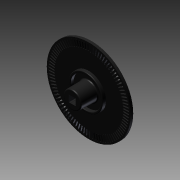
# Autodesk Inventor part: 276-2156
Saved by Autodesk Inventor 2013 (Build 170138000, 138)
## iProperties
Category: Sensors
Company: Autodesk Inc.
Created: 2012-04-06
Part Number: 276-2156
Document SubType Name: Modeling
Designer: Autodesk Inc.
Density: 1 g/cm^3
Catalog Web Link: http://www.vexrobotics.com/276-2156.html
Vendor: VEX
Material: Generic
Author: Autodesk Inc.
Autodesk Inventor part; units mm, degrees
ref_plane "YZ Plane" through (0, 0, 0) normal (1, 0, 0) x (0, 1, 0)
ref_plane "XZ Plane" through (0, 0, 0) normal (0, 1, 0) x (-1, 0, 0)
ref_plane "XY Plane" through (0, 0, 0) normal (0, 0, 1) x (1, 0, 0)
sketch "Sketch1" plane through (0, 0, 0) normal (0, 0, 1) x (1, 0, 0)
  circle A0 centre (0, 0) radius 20.0025
  dimension "d0" = 40.005
  constraints: 1 centre point, 1 coincident
  measures "d0" diameter of A0
extrude "Extrusion1" add sketch "Sketch1" along normal mid plane 1.2446
sketch "Sketch2" plane through (0, 0, 0.6223) normal (0, 0, 1) x (1, 0, 0)
  circle A0 centre (0, 0) radius 20.0025 projected
  circle A1 centre (0, 0) radius 4.3187
  dimension "d3" = 8.6374
  constraints: 1 centre point, 1 coincident
  measures "d3" diameter of A1
extrude "Extrusion2" add sketch "Sketch2" along normal blind 7.874 draft -0.5 contours A1
fillet "Fillet1" radius 0.508 2 edges at (-4.3187, 0, 0.6223) (-4.25, 0, 8.4963)
sketch "Sketch3" plane through (0, 0, 0.6223) normal (0, 0, 1) x (1, 0, 0)
  circle A0 centre (0, 0) radius 4.8223 projected
  circle A1 centre (0, 0) radius 7.2238
  circle A2 centre (0, 0) radius 8.2652
  dimension "d7" = 14.4476
  dimension "d8" = 1.0414
  constraints: 2 centre point, 2 coincident
  measures "d7" diameter of A1
  measures "d8" radial gap between concentric circles of A2 A1
extrude "Extrusion3" add sketch "Sketch3" along normal blind 1.4986 draft -1 contours A2
fillet "Fillet2" radius 0.3048 2 edges at (-8.2391, 0, 2.1209) (-7.25, 0, 2.1209)
mirror "Mirror1" about plane through (0, 0, 0) normal (0, 0, 1) of "Extrusion1", "Extrusion2", "Fillet1"
sketch "Sketch4" plane through (0, 0, 8.4963) normal (0, 0, 1) x (1, 0, 0)
  ellipse E0 centre (0.0646, -0.7293) end of major axis (-2.4878, -3.9719) minor radius 3.3908 (3.7543, 0.0005) -> (3.7536, 0.0771) ccw
  spline S0 degree 3 poles (3.7536, 0.0771) (3.7488, 0.3133) (3.7224, 0.5454) (3.6744, 0.7733) (3.6504, 0.8873) (3.6209, 1.0002) (3.5861, 1.1121) (3.5512, 1.224) (3.5122, 1.3325) (3.4637, 1.4484) (3.3668, 1.6803) (3.2489, 1.8987) (3.1046, 2.111) (2.9603, 2.3234) (2.7944, 2.5203) (2.6099, 2.6988) (2.5176, 2.7881) (2.4212, 2.8723) (2.3205, 2.9514) (2.2198, 3.0306) (2.1131, 3.1057) (2.0069, 3.1729) (1.9007, 3.2401) (1.7915, 3.3018) (1.6793, 3.3579) (1.6232, 3.3859) (1.5664, 3.4126) (1.5088, 3.4378) (1.4512, 3.4631) (1.3921, 3.4872) (1.3369, 3.5083) (1.116, 3.5926) (0.8909, 3.6552) (0.6616, 3.6962) (0.4323, 3.7372) (0.1977, 3.7565) (-0.0388, 3.7542) (-0.2753, 3.7518) (-0.5078, 3.7278) (-0.7362, 3.6821) (-0.8504, 3.6592) (-0.9635, 3.6309) (-1.0757, 3.5972) (-1.1318, 3.5804) (-1.1876, 3.5622) (-1.2432, 3.5426) (-1.2988, 3.523) (-1.3525, 3.5028) (-1.4108, 3.4792) (-1.5273, 3.432) (-1.6411, 3.3791) (-1.752, 3.3206) (-1.8629, 3.262) (-1.9695, 3.1988) (-2.0766, 3.1278) (-2.2906, 2.9857) (-2.4891, 2.8223) (-2.6698, 2.6396) (-2.7601, 2.5483) (-2.8454, 2.4527) (-2.9256, 2.3529) (-2.9658, 2.303) (-3.0046, 2.252) (-3.0422, 2.2) (-3.0798, 2.148) (-3.1168, 2.094) (-3.151, 2.0412) (-3.2194, 1.9356) (-3.2823, 1.827) (-3.3395, 1.7155) (-3.3682, 1.6597) (-3.3954, 1.6032) (-3.4213, 1.546) (-3.4342, 1.5173) (-3.4468, 1.4885) (-3.459, 1.4595) (-3.4713, 1.4305) (-3.4836, 1.4001) (-3.4945, 1.3725) (-3.6677, 0.9317) (-3.7543, 0.474) (-3.7543, -0.0005) knots 0.006695 0.006695 0.006695 0.006695 0.068777 0.068777 0.068777 0.099817 0.099817 0.099817 0.130858 0.130858 0.130858 0.19294 0.19294 0.19294 0.255021 0.255021 0.255021 0.286062 0.286062 0.286062 0.317103 0.317103 0.317103 0.348144 0.348144 0.348144 0.363664 0.363664 0.363664 0.379184 0.379184 0.379184 0.441266 0.441266 0.441266 0.503348 0.503348 0.503348 0.565429 0.565429 0.565429 0.59647 0.59647 0.59647 0.61199 0.61199 0.61199 0.627511 0.627511 0.627511 0.658551 0.658551 0.658551 0.689592 0.689592 0.689592 0.751674 0.751674 0.751674 0.782715 0.782715 0.782715 0.798235 0.798235 0.798235 0.813755 0.813755 0.813755 0.844796 0.844796 0.844796 0.860316 0.860316 0.860316 0.868077 0.868077 0.868077 0.875837 0.875837 0.875837 1 1 1 1
  arc A0 (-3.7543, -0.0005) -> (-3.7536, -0.0771) centre (0, 0) ccw
  spline S1 degree 3 poles (-3.7536, -0.0771) (-3.7488, -0.3133) (-3.7224, -0.5454) (-3.6744, -0.7733) (-3.6504, -0.8873) (-3.6209, -1.0002) (-3.5861, -1.1121) (-3.5512, -1.224) (-3.5122, -1.3324) (-3.4637, -1.4484) (-3.3668, -1.6803) (-3.2489, -1.8987) (-3.1046, -2.111) (-2.9603, -2.3234) (-2.7944, -2.5203) (-2.6099, -2.6988) (-2.5176, -2.7881) (-2.4212, -2.8723) (-2.3205, -2.9514) (-2.2198, -3.0306) (-2.1131, -3.1057) (-2.0069, -3.1729) (-1.9007, -3.2401) (-1.7915, -3.3018) (-1.6793, -3.3579) (-1.6232, -3.3859) (-1.5664, -3.4126) (-1.5088, -3.4378) (-1.4512, -3.4631) (-1.3921, -3.4872) (-1.3369, -3.5083) (-1.116, -3.5926) (-0.8909, -3.6552) (-0.6616, -3.6962) (-0.4323, -3.7372) (-0.1977, -3.7565) (0.0388, -3.7541) (0.2753, -3.7518) (0.5078, -3.7278) (0.7362, -3.6821) (0.8504, -3.6592) (0.9636, -3.6309) (1.0757, -3.5972) (1.1318, -3.5804) (1.1876, -3.5622) (1.2432, -3.5426) (1.2988, -3.523) (1.3525, -3.5028) (1.4108, -3.4792) (1.5273, -3.432) (1.6411, -3.3791) (1.752, -3.3205) (1.8629, -3.262) (1.9695, -3.1988) (2.0766, -3.1278) (2.2906, -2.9857) (2.4891, -2.8223) (2.6698, -2.6396) (2.7601, -2.5482) (2.8454, -2.4527) (2.9256, -2.3529) (2.9658, -2.303) (3.0046, -2.252) (3.0422, -2.2) (3.0798, -2.148) (3.1168, -2.094) (3.151, -2.0412) (3.2194, -1.9356) (3.2823, -1.827) (3.3395, -1.7155) (3.3682, -1.6597) (3.3954, -1.6032) (3.4213, -1.546) (3.4342, -1.5173) (3.4468, -1.4885) (3.459, -1.4595) (3.4713, -1.4305) (3.4836, -1.4001) (3.4945, -1.3725) (3.6677, -0.9317) (3.7543, -0.474) (3.7543, 0.0005) knots 0.006695 0.006695 0.006695 0.006695 0.068776 0.068776 0.068776 0.099817 0.099817 0.099817 0.130858 0.130858 0.130858 0.192939 0.192939 0.192939 0.255021 0.255021 0.255021 0.286062 0.286062 0.286062 0.317102 0.317102 0.317102 0.348143 0.348143 0.348143 0.363664 0.363664 0.363664 0.379184 0.379184 0.379184 0.441266 0.441266 0.441266 0.503347 0.503347 0.503347 0.565429 0.565429 0.565429 0.59647 0.59647 0.59647 0.61199 0.61199 0.61199 0.62751 0.62751 0.62751 0.658551 0.658551 0.658551 0.689592 0.689592 0.689592 0.751674 0.751674 0.751674 0.782714 0.782714 0.782714 0.798235 0.798235 0.798235 0.813755 0.813755 0.813755 0.844796 0.844796 0.844796 0.860316 0.860316 0.860316 0.868077 0.868077 0.868077 0.875837 0.875837 0.875837 1 1 1 1
  line L0 (1.6128, 0.8257) -> (1.5674, 0.8812)
  line L1 (1.6128, 0.8257) -> (1.613, -0.8253)
  line L2 (1.5676, -0.8807) -> (1.613, -0.8253)
  arc A1 (1.5676, -0.8807) -> (1.5676, -0.8968) centre (1.5775, -0.8888) ccw
  line L3 (1.613, -0.9523) -> (1.5676, -0.8968)
  line L4 (1.613, -0.9523) -> (1.6131, -1.6127)
  line L5 (1.6131, -1.6127) -> (0.9527, -1.6128)
  line L6 (0.8973, -1.5674) -> (0.9527, -1.6128)
  arc A2 (0.8973, -1.5674) -> (0.8812, -1.5674) centre (0.8892, -1.5772) ccw
  line L7 (0.8257, -1.6128) -> (0.8812, -1.5674)
  line L8 (0.8257, -1.6128) -> (-0.8253, -1.613)
  line L9 (-0.8807, -1.5676) -> (-0.8253, -1.613)
  arc A3 (-0.8807, -1.5676) -> (-0.8968, -1.5676) centre (-0.8888, -1.5775) ccw
  line L10 (-0.9523, -1.613) -> (-0.8968, -1.5676)
  line L11 (-0.9523, -1.613) -> (-1.6127, -1.6131)
  line L12 (-1.6127, -1.6131) -> (-1.6128, -0.9527)
  line L13 (-1.5674, -0.8973) -> (-1.6128, -0.9527)
  arc A4 (-1.5674, -0.8973) -> (-1.5674, -0.8812) centre (-1.5772, -0.8892) ccw
  line L14 (-1.6128, -0.8257) -> (-1.5674, -0.8812)
  line L15 (-1.6128, -0.8257) -> (-1.613, 0.8253)
  line L16 (-1.5676, 0.8807) -> (-1.613, 0.8253)
  arc A5 (-1.5676, 0.8807) -> (-1.5676, 0.8968) centre (-1.5775, 0.8888) ccw
  line L17 (-1.613, 0.9523) -> (-1.5676, 0.8968)
  line L18 (-1.613, 0.9523) -> (-1.6131, 1.6127)
  line L19 (-1.6131, 1.6127) -> (-0.9527, 1.6128)
  line L20 (-0.8973, 1.5674) -> (-0.9527, 1.6128)
  arc A6 (-0.8973, 1.5674) -> (-0.8812, 1.5674) centre (-0.8892, 1.5772) ccw
  line L21 (-0.8812, 1.5674) -> (-0.8257, 1.6128)
  line L22 (-0.8257, 1.6128) -> (0.8253, 1.613)
  line L23 (0.8807, 1.5676) -> (0.8253, 1.613)
  arc A7 (0.8807, 1.5676) -> (0.8968, 1.5676) centre (0.8888, 1.5775) ccw
  line L24 (0.9523, 1.613) -> (0.8968, 1.5676)
  line L25 (0.9523, 1.613) -> (1.6127, 1.6131)
  line L26 (1.6127, 1.6131) -> (1.6128, 0.9527)
  line L27 (1.5674, 0.8973) -> (1.6128, 0.9527)
  arc A8 (1.5674, 0.8973) -> (1.5674, 0.8812) centre (1.5772, 0.8892) ccw
  constraints: 56 end point, 18 point on circle, 9 centre point, 8 other
extrude "Extrusion4" cut sketch "Sketch4" against normal up to next contours L1 L2 A1 L3 L4 L5 L6 A2 L7 L8 L9 A3 L10 L11 L12 L13 A4 L14 L15 L16 A5 L17 L18 L19 L20 A6 L21 L22 L23 A7 L24 L25 L26 L27 A8 L0
sketch "Sketch5" plane through (0, 0, 0.6223) normal (0, 0, 1) x (1, 0, 0)
  arc A0 (-0.0816, 19.0015) -> (-0.5816, 18.9927) centre (-0.3316, 18.9971) ccw
  line L0 (-0.0816, 19.0015) -> (-0.038, 16.5019)
  arc A1 (-0.5379, 16.4931) -> (-0.038, 16.5019) centre (-0.288, 16.4975) ccw
  line L1 (-0.5379, 16.4931) -> (-0.5816, 18.9927)
  line L2 (0, 0) -> (0, 20) construction
  line L3 (0, 0) -> (-0.288, 16.4975) construction
  constraints: 8 end point, 4 point on circle, 2 centre point, 1 parallel, 1 vertical
extrude "Extrusion5" cut sketch "Sketch5" against normal up to next
pattern_circular "Circular Pattern1" count 90 over 360 about axis through (0, 0, 0.6223) along (0, 0, 1) of "Extrusion5"
sketch "Sketch6" plane through (0, 0, 8.4963) normal (0, 0, 1) x (1, 0, 0)
  line L0 (1.6128, 0.8257) -> (1.613, -0.8253) projected
  line L1 (0.8257, -1.6128) -> (-0.8253, -1.613) projected
  line L2 (-1.6128, -0.8257) -> (-1.613, 0.8253) projected
  line L3 (-0.8257, 1.6128) -> (0.8253, 1.613) projected
  circle A0 centre (0, 0) radius 3.7464 projected
  circle A1 centre (0, 0) radius 1.6129
  constraints: 4 tangent, 1 centre point, 1 coincident
surface extrude "ExtrusionSrf1" sketch "Sketch6" against normal up to surface (16.9926 mm away) shown no curves A1
body "Solid1"
body "Srf1"
